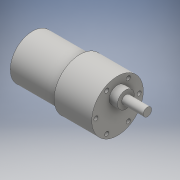
# Autodesk Inventor part: SPG30_Motor
Saved by Autodesk Inventor 2016 (Build 200138000, 138)
## iProperties
Created: 2016-01-06
Part Number: SPG30_Motor
Material: Generic
Document SubType Name: Modeling
Designer: m2memari
Density: 1 g/cm^3
Appearance: Default
Author: m2memari
Autodesk Inventor part; units mm, degrees
ref_plane "YZ Plane" through (0, 0, 0) normal (1, 0, 0) x (0, 1, 0)
ref_plane "XZ Plane" through (0, 0, 0) normal (0, 1, 0) x (-1, 0, 0)
ref_plane "XY Plane" through (0, 0, 0) normal (0, 0, 1) x (1, 0, 0)
sketch "Sketch1" plane through (0, 0, 0) normal (1, 0, 0) x (0, 1, 0)
  circle A0 centre (0, 0) radius 18.5
  dimension "d0" = 37
  constraints: 1 centre point, 1 coincident
  measures "d0" diameter of A0
extrude "Extrusion1" add sketch "Sketch1" along normal blind 27
sketch "Sketch2" plane through (0, 0, 0) normal (-1, 0, 0) x (0, 0, 1)
  circle A0 centre (0, 0) radius 16
  dimension "d3" = 32
  constraints: 1 centre point, 1 coincident
  measures "d3" diameter of A0
extrude "Extrusion2" add sketch "Sketch2" along normal blind 34
sketch "Sketch3" plane through (27, 0, 0) normal (1, 0, 0) x (0, 0, -1)
  circle A0 centre (0, 15.5) radius 1.5
  circle A1 centre (-13.4234, 7.75) radius 1.5
  circle A2 centre (-13.4234, -7.75) radius 1.5
  circle A3 centre (0, -15.5) radius 1.5
  circle A4 centre (13.4234, -7.75) radius 1.5
  circle A5 centre (13.4234, 7.75) radius 1.5
  point P0 (0, 0)
  dimension "d8" = 3
  dimension "d9" = 15.5
  dimension "d12" = 360
  constraints: 6 centre point, 1 vertical alignment, 13 other
  measures "d8" diameter of A0
  measures "d9" distance of point (0, 0) A0.centre
extrude "Extrusion3" cut sketch "Sketch3" against normal blind 3
sketch "Sketch4" plane through (27, 0, 0) normal (1, 0, 0) x (0, 0, -1)
  circle A0 centre (-7, 0) radius 6
  point P0 (0, 0)
  dimension "d16" = 12
  dimension "d17" = 7
  constraints: 1 centre point, 1 horizontal alignment
  measures "d16" diameter of A0
  measures "d17" distance of point (0, 0) A0.centre
extrude "Extrusion4" add sketch "Sketch4" along normal blind 6
sketch "Sketch5" plane through (33, 0, 7) normal (1, 0, 0) x (0, 0, -1)
  circle A0 centre (0, 0) radius 3
  point P0 (7, 0)
  dimension "d20" = 6
  dimension "d21" = 7
  constraints: 1 centre point, 1 horizontal alignment
  measures "d20" diameter of A0
  measures "d21" distance of point (7, 0) A0.centre
extrude "Extrusion5" add sketch "Sketch5" along normal blind 15.5
body "Solid1"
